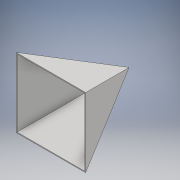
# Autodesk Inventor part: pyramid
Saved by Autodesk Inventor 2018 (Build 220112000, 112)
## iProperties
Created: 2019-03-14
Part Number: pyramid
Material: Generic
Document SubType Name: Modeling
Designer: hryst
Density: 1 g/cm^3
Appearance: Default
Author: hryst
Autodesk Inventor part; units mm, degrees
ref_plane "YZ Plane" through (0, 0, 0) normal (1, 0, 0) x (0, 1, 0)
ref_plane "XY Plane" through (0, 0, 0) normal (0, 0, 1) x (1, 0, 0)
sketch "Sketch1" plane through (0, 0, 0) normal (0, 1, 0) x (-1, 0, 0)
  line L0 (-80, 80) -> (80, 80)
  line L1 (80, 80) -> (80, -80)
  line L2 (80, -80) -> (-80, -80)
  line L3 (-80, -80) -> (-80, 80)
  line L4 (-80, 80) -> (80, -80) construction
  line L5 (80, 80) -> (-80, -80) construction
  point P0 (0, 0)
  dimension "d0" = 160
  dimension "d1" = 160
  constraints: 12 end point, 2 midpoint, 2 parallel, 1 horizontal, 1 perpendicular
  measures "d0" distance of L1.end L2.end
  measures "d1" distance of L0.end L1.end
ref_plane "Work Plane3" through (0, 180, 0) normal (0, 1, 0) x (-1, 0, 0)
sketch "Sketch7" plane through (0, 180, 0) normal (0, 1, 0) x (-1, 0, 0)
  point P0 (0, 0)
  point P1 (0, 0)
  constraints: 1 coincident
loft "Loft2" add profiles "Sketch1" section 2 point at (0, 180, 0)
shell "Shell2" thickness 2 removed faces 1 at (26.6667, 0, 26.6667)
body "Solid2"
